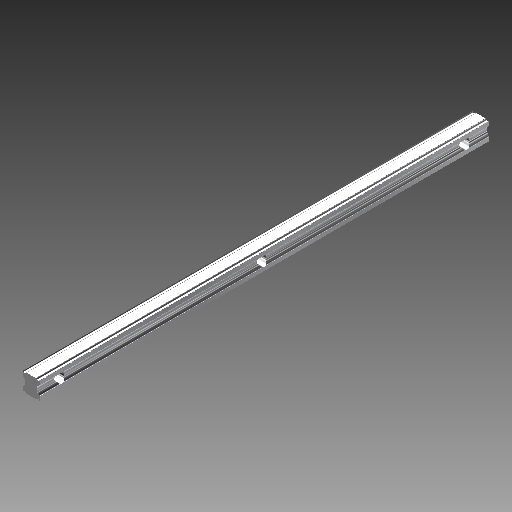
# Autodesk Inventor part: SAR330-30_r
Saved by Autodesk Inventor 2019 (Build 230136000, 136)
## iProperties
Category: PARTsolutions
Company: MISUMI
Created: 2019-04-19
Part Number: SAR330-30_r
Material: Aluminum 6061
Catalog Web Link: www.cadenas.de
Description: SAR3_rail-Slide Rails - Aluminum Alloy - Three - Step Slide Rails
Vendor: MISUMI
Document SubType Name: Modeling
Designer: psadmin
Manufacturer: MISUMI
Mass: 89.3851 g
Surface Area: 157.859 cm^2
Volume: 33.1056 cm^3
Density: 2.7 g/cm^3
Appearance: Aluminum - Flat
PSOL_IDENT_0: {$CADENAS_DATA\23d-libs\misumi\metric\07_slide_rails\sar3_series\sar3_rail.prj},167 {VTYP=3D},{NB=SA
PSOL_IDENT_1: R330-30_r},{LINA=SAR330-30},{NN=SAR3_rail},{DATE=30.03.2018 01:39:43},{GEOMDATE=15.05.2017 01:02:00}
PSOL_IDENT_2: ,{VERSION=},{LINEID=10},{WBVAR=NO},{WBNUMERIC=NO}  {NB=SAR330-30_r},{LINA=SAR330-30},{KT=DUMMY},{PN=
PSOL_IDENT_3: SAR330-30},{TYPE=SAR330},{MAT1=Aluminum Alloy},{ST1=Clear Anodizing},{MAT2=Aluminum Alloy},{ST2=Clea
PSOL_IDENT_4: r Anodizing},{MAT3=Steel},{NO=30},{RL=300},{TD=345},{A=135},{B=270},{C=135},{D=270},{RLO=147},{BA=25
PSOL_IDENT_5: },{PPATH=sar3_series\\sar3_templ.prj}
NN: SAR3_rail
NT: Slide Rails - Aluminum Alloy - Three - Step Slide Rails
NB: SAR330-30_r
NBSYN: $PN._r
LINA: SAR330-30
PN: SAR330-30
MAT1: Aluminum Alloy
ST1: Clear Anodizing
MAT2: Aluminum Alloy
ST2: Clear Anodizing
MAT3: Steel
NO: 30
RLO: 147
SUPPLIER: MISUMI
ARTICLENO: SAR330-30_r
BOMINFO: SAR330-30
CREATOR: CADENAS GmbH
Title: SAR330-30
Author: Cadenas PARTsolutions
Comments: Slide Rails - Aluminum Alloy - Three - Step Slide Rails
Autodesk Inventor part; units mm, degrees
sketch "Sketch_1" plane through (0, 0, 0) normal (0, 0, 1) x (1, 0, 0)
  line L0 (0, 2.9516) -> (0, 0.3457)
  arc A0 (2.6416, 0) -> (0, 0.3457) centre (1.2, -0.75) ccw
  line L1 (2.6416, 0) -> (8.7584, 0)
  arc A1 (11.4, 0.3457) -> (8.7584, 0) centre (10.2, -0.75) ccw
  line L2 (11.4, 0.3457) -> (11.4, 2.9516)
  arc A2 (11.4, 9.1484) -> (11.4, 2.9516) centre (12.8, 6.05) ccw
  line L3 (11.4, 9.1484) -> (11.4, 11.7543)
  arc A3 (8.7584, 12.1) -> (11.4, 11.7543) centre (10.2, 12.85) ccw
  line L4 (8.7584, 12.1) -> (2.6416, 12.1)
  arc A4 (0, 11.7543) -> (2.6416, 12.1) centre (1.2, 12.85) ccw
  line L5 (0, 11.7543) -> (0, 9.1484)
  arc A5 (0, 2.9516) -> (0, 9.1484) centre (-1.4, 6.05) ccw
  constraints: 12 end point, 12 point on circle, 6 centre point
extrude "Extrusion1" add sketch "Sketch_1" along normal blind 300
sketch "Sketch_3" plane through (0, 0, 15) normal (0, 0, 1) x (1, 0, 0)
  line L0 (11.4, 6.05) -> (0, 6.05)
  line L1 (0, 6.05) -> (0, 9.3)
  line L2 (0, 9.3) -> (11.4, 9.3)
  line L3 (11.4, 9.3) -> (11.4, 6.05)
  line L4 (11.4, 6.05) -> (0, 6.05)
  constraints: 10 end point
revolve "Revolution1" cut sketch "Sketch_3" angle 360 about axis through (11.4, 6.05, 15) along (1, 0, 0)
pattern_linear "Rectangular Pattern1" count 3 spacing 135 along (0, 0, 1) of "Revolution1"
ref_plane "to_ball_1_XY" through (1.2, -0.75, 109.375) normal (0, 0, 1) x (1, 0, 0)
ref_plane "to_ball_1_YZ" through (1.2, -0.75, 109.375) normal (1, 0, 0) x (0, 1, 0)
ref_plane "to_ball_1_ZX" through (1.2, -0.75, 109.375) normal (0, 1, 0) x (0, 0, 1)
ref_plane "to_ball_2_XY" through (10.2, -0.75, 109.375) normal (0, 0, 1) x (1, 0, 0)
ref_plane "to_ball_2_YZ" through (10.2, -0.75, 109.375) normal (1, 0, 0) x (0, 1, 0)
ref_plane "to_ball_2_ZX" through (10.2, -0.75, 109.375) normal (0, 1, 0) x (0, 0, 1)
ref_plane "to_ball_3_XY" through (1.2, 12.85, 109.375) normal (0, 0, 1) x (1, 0, 0)
ref_plane "to_ball_3_YZ" through (1.2, 12.85, 109.375) normal (1, 0, 0) x (0, 1, 0)
ref_plane "to_ball_3_ZX" through (1.2, 12.85, 109.375) normal (0, 1, 0) x (0, 0, 1)
ref_plane "to_ball_4_XY" through (10.2, 12.85, 109.375) normal (0, 0, 1) x (1, 0, 0)
ref_plane "to_ball_4_YZ" through (10.2, 12.85, 109.375) normal (1, 0, 0) x (0, 1, 0)
ref_plane "to_ball_4_ZX" through (10.2, 12.85, 109.375) normal (0, 1, 0) x (0, 0, 1)
ref_plane "to_body_XY" through (5.6, 6.05, 150) normal (0, 0, 1) x (1, 0, 0)
ref_plane "to_body_YZ" through (5.6, 6.05, 150) normal (1, 0, 0) x (0, 1, 0)
ref_plane "to_body_ZX" through (5.6, 6.05, 150) normal (0, 1, 0) x (0, 0, 1)
ref_plane "to_body2_XY" through (5.8, 6.05, 150) normal (0, 0, 1) x (1, 0, 0)
ref_plane "to_body2_YZ" through (5.8, 6.05, 150) normal (1, 0, 0) x (0, 1, 0)
ref_plane "to_body2_ZX" through (5.8, 6.05, 150) normal (0, 1, 0) x (0, 0, 1)
body "Solid1"
